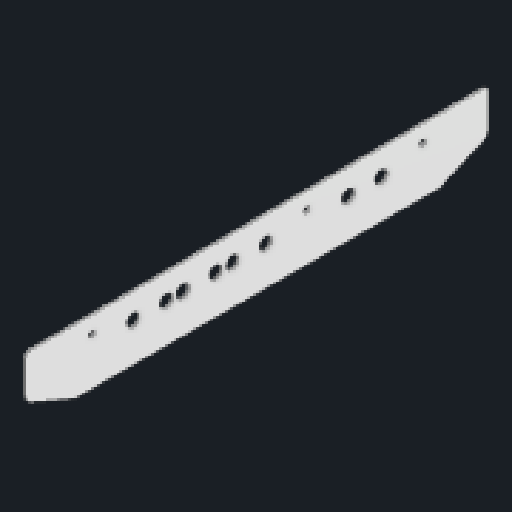
# Autodesk Inventor part: Skirt
Saved by Autodesk Inventor 2025 (Build 290162000, 162)
## iProperties
Created: 2025-01-27
Part Number: Skirt
Material: Acetal Resin, White
Document SubType Name: Modeling
Designer: Averey Ku
Density: 1.425 g/cm^3
Appearance: Smooth - White
Author: Averey Ku
Autodesk Inventor part; units mm, degrees
ref_plane "YZ Plane" through (0, 0, 0) normal (1, 0, 0) x (0, 1, 0)
ref_plane "XZ Plane" through (0, 0, 0) normal (0, 1, 0) x (-1, 0, 0)
ref_plane "XY Plane" through (0, 0, 0) normal (0, 0, 1) x (1, 0, 0)
sketch "skirt" plane through (0, 0, 0) normal (0, 0, 1) x (1, 0, 0)
  circle A0 centre (5.0031, 25.9038) radius 4.7625
  line L0 (24.0531, -167.7712) -> (24.0531, 181.4788)
  line L1 (-25.1594, 145.2504) -> (-25.1594, -131.5428)
  circle A1 centre (11.3531, 133.8538) radius 2.1844
  arc A2 (24.0531, 181.4788) -> (20.8781, 184.6538) centre (20.8781, 181.4788) ccw
  line L2 (20.8781, 184.6538) -> (-4.6437, 184.6538)
  line L3 (-24.646, 147.7518) -> (-10.4803, 180.8052)
  arc A3 (-4.6437, 184.6538) -> (-10.4803, 180.8052) centre (-4.6437, 178.3038) ccw
  arc A4 (-24.646, 147.7518) -> (-25.1594, 145.2504) centre (-18.8094, 145.2504) ccw
  line L4 (-24.646, -134.0442) -> (-10.4803, -167.0976)
  line L5 (-4.6437, -170.9462) -> (20.8781, -170.9462)
  arc A5 (20.8781, -170.9462) -> (24.0531, -167.7712) centre (20.8781, -167.7712) ccw
  arc A6 (-25.1594, -131.5428) -> (-24.646, -134.0442) centre (-18.8094, -131.5428) ccw
  circle A7 centre (11.3531, -120.1462) radius 2.1844
  arc A8 (-10.4803, -167.0976) -> (-4.6437, -170.9462) centre (-4.6437, -164.5962) ccw
  circle A9 centre (5.0031, 102.1038) radius 4.7625
  circle A10 centre (5.0031, 76.7038) radius 4.7625
  circle A11 centre (5.0031, 64.0038) radius 4.7625
  circle A12 centre (5.0031, 38.6038) radius 4.7625
  circle A13 centre (5.0031, 0.5038) radius 4.7625
  circle A14 centre (11.3531, -31.2462) radius 2.1844
  circle A15 centre (5.0031, -62.9962) radius 4.7625
  circle A16 centre (5.0031, -88.3962) radius 4.7625
  point P0 (-0.9322, -0.2017)
  point P1 (5.0031, 51.3038)
  point P2 (-25.1594, 146.5538)
  point P3 (-25.1594, -132.8462)
  point P4 (5.0031, -12.1962)
  point P5 (5.0031, 13.2038)
  dimension "d0" = 279.4
  dimension "d1" = 49.2125
  dimension "d2" = 3.175
  dimension "d3" = 113.199
  dimension "d4" = 113.199
  dimension "d5" = 6.35
  dimension "d7" = 9.525
  dimension "d13" = 50.8
  dimension "d14" = 50.8
  dimension "d15" = 9.525
  dimension "d16" = 4.3688
  dimension "d17" = 31.75
  measures "d0" distance of point (-25.159, 146.554) point (-25.159, -132.846)
  measures "d1" distance between parallel lines of L0 L1
  measures "d2" radius of A2
  measures "d3" angle of L2 L3
  measures "d4" angle of L5 L4
  measures "d5" radius of A3
  measures "d7" diameter of A0
  measures "d13" distance from line of A1.centre L2
  measures "d14" distance from line of A7.centre L5
  measures "d15" diameter of A9
  measures "d16" diameter of A14
  measures "d17" vertical distance of A16.centre A7.centre
sketch "Sketch1" plane through (0, 0, 0) normal (1, 0, 0) x (0, 1, 0)
  circle A0 centre (-6.35, -107.95) radius 4.7625
  line L0 (12.7, -301.625) -> (12.7, 47.625)
  line L1 (-36.5125, 11.3966) -> (-36.5125, -265.3966)
  circle A1 centre (0, 0) radius 2.1844
  arc A2 (12.7, 47.625) -> (9.525, 50.8) centre (9.525, 47.625) ccw
  line L2 (9.525, 50.8) -> (-15.9968, 50.8)
  line L3 (-35.9991, 13.898) -> (-21.8333, 46.9514)
  arc A3 (-15.9968, 50.8) -> (-21.8333, 46.9514) centre (-15.9968, 44.45) ccw
  arc A4 (-35.9991, 13.898) -> (-36.5125, 11.3966) centre (-30.1625, 11.3966) ccw
  line L4 (-35.9991, -267.898) -> (-21.8333, -300.9514)
  line L5 (-15.9968, -304.8) -> (9.525, -304.8)
  arc A5 (9.525, -304.8) -> (12.7, -301.625) centre (9.525, -301.625) ccw
  arc A6 (-36.5125, -265.3966) -> (-35.9991, -267.898) centre (-30.1625, -265.3966) ccw
  circle A7 centre (0, -254) radius 2.1844
  arc A8 (-21.8333, -300.9514) -> (-15.9968, -304.8) centre (-15.9968, -298.45) ccw
  circle A9 centre (-6.35, -31.75) radius 4.7625
  circle A10 centre (-6.35, -57.15) radius 4.7625
  circle A11 centre (-6.35, -69.85) radius 4.7625
  circle A12 centre (-6.35, -95.25) radius 4.7625
  circle A13 centre (-6.35, -133.35) radius 4.7625
  circle A14 centre (0, -165.1) radius 2.1844
  circle A15 centre (-6.35, -196.85) radius 4.7625
  circle A16 centre (-6.35, -222.25) radius 4.7625
  constraints: 1 other
extrude "Extrusion1" add sketch "Sketch1" along normal blind 1.5875
body "Solid1"
